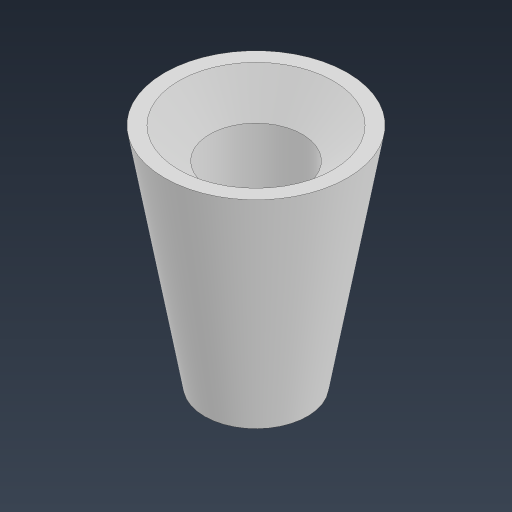
# Autodesk Inventor part: holder_for_felgen
Saved by Autodesk Inventor 2023 (Build 270158000, 158)
## iProperties
Created: 2026-02-19
Part Number: holder_for_felgen
Material: Generic
Document SubType Name: Modeling
Designer: szymo
Density: 1 g/cm^3
Appearance: Default
Author: szymo
Autodesk Inventor part; units mm, degrees
ref_plane "YZ Plane" through (0, 0, 0) normal (1, 0, 0) x (0, 1, 0)
ref_plane "XZ Plane" through (0, 0, 0) normal (0, 1, 0) x (-1, 0, 0)
ref_plane "XY Plane" through (0, 0, 0) normal (0, 0, 1) x (1, 0, 0)
sketch "Sketch1" plane through (0, 0, 0) normal (1, 0, 0) x (0, 1, 0)
  line L0 (0, 0) -> (0, 3.5527)
  line L1 (0, 3.5527) -> (-8.8055, 2)
  line L2 (-8.8055, 2) -> (-8.8055, 0)
  line L3 (-8.8055, 0) -> (0, 0)
  line L4 (-2, 3.2) -> (-12.3498, 3.2) construction
  line L5 (-12.3498, 3.2) -> (-12.3498, 0) construction
  line L6 (-12.3498, 0) -> (-8.8055, 0) construction
  dimension "d0" = 2
  dimension "d1" = 100
  dimension "d2" = 3.2
  dimension "d12" = 2
  constraints: 14 end point, 2 horizontal, 2 point on line, 1 collinear, 1 parallel, 1 perpendicular, 1 vertical
  measures "d0" distance of L1.end L2.end
  measures "d1" angle of L1 L2
  measures "d2" distance between parallel lines of L4 L6
  measures "d12" distance from line of L0 L4.start
revolve "Revolution1" add sketch "Sketch1" angle 360 about axis through (0, -8.8055, 0) along (0, 1, 0)
sketch "Sketch2" plane through (0, 0, 0) normal (0, 1, 0) x (1, 0, 0)
  circle A0 centre (0, 0) radius 3.5527 projected
hole "Hole1" at (0, 0, 0) direction (0, -1, 0) diameter 3.6 end through all countersink diameter 6 countersink angle 90 clearance for "Countersunk Flat Head Screw ISO 2009/7046" size "M3" standard "ISO"
body "Solid1"
